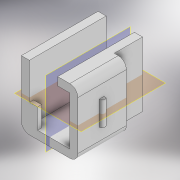
# Autodesk Inventor part: 부품1
Saved by Autodesk Inventor 2020 (Build 240168000, 168)
## iProperties
Created: 2022-04-05
Part Number: 부품1
Material: 일반
Document SubType Name: Modeling
Designer: Knowblesse
Density: 1 g/cm^3
Appearance: 기본값
Author: Knowblesse
## iProperties of the stored document _3D 인쇄.ipt
Created: 2022-04-05
Part Number: _3D 인쇄
Material: 일반
Document SubType Name: Modeling
Designer: Knowblesse
Density: 1 g/cm^3
Appearance: 기본값
Author: Knowblesse
Autodesk Inventor part; units mm, degrees
ref_plane "YZ Plane" through (0, 0, 0) normal (1, 0, 0) x (0, 1, 0)
ref_plane "XZ Plane" through (0, 0, 0) normal (0, 1, 0) x (-1, 0, 0)
ref_plane "XY Plane" through (0, 0, 0) normal (0, 0, 1) x (1, 0, 0)
sketch "스케치1" plane through (0, 0, 0) normal (0, 0, 1) x (1, 0, 0)
  line L0 (-3.5, -6) -> (3.5, -6)
  line L1 (3.5, -6) -> (3.5, 6)
  line L2 (3.5, 6) -> (-3.5, 6)
  line L3 (-3.5, 6) -> (-3.5, -6)
  line L4 (-3.5, -6) -> (3.5, 6) construction
  line L5 (3.5, -6) -> (-3.5, 6) construction
  line L6 (-5.5, 8) -> (-5.5, -8)
  line L7 (-5.5, -8) -> (5.5, -8)
  line L8 (5.5, -8) -> (5.5, 8)
  line L9 (5.5, 8) -> (3.5, 8)
  line L10 (3.5, 8) -> (3.5, 6)
  line L11 (-5.5, 8) -> (-3.5, 8)
  line L12 (-3.5, 8) -> (-3.5, 6)
  point P0 (0, 0)
  dimension "d0" = 7
  dimension "d1" = 12
  dimension "d2" = 2
  dimension "t" = 2
  dimension "d4" = 2
  dimension "d5" = 2
  constraints: 26 end point, 6 perpendicular, 2 midpoint, 2 parallel, 1 horizontal, 1 point on line, 1 vertical
  measures "d0" distance of L2.end L1.end
  measures "d1" distance of L1.end L0.end
  measures "d2" distance between parallel lines of L3 L6
  measures "t" distance between parallel lines of L8 L1
  measures "d4" distance between parallel lines of L0 L7
  measures "d5" distance between parallel lines of L11 L2
extrude "돌출1" add sketch "스케치1" along normal blind 7 contours L0 L1 L10 L9 L8 L7 L6 L11 L12 L3
sketch "스케치2" plane through (0, 0, 7) normal (0, 0, 1) x (1, 0, 0)
  line L0 (3.5, 8) -> (3.5, -6) projected
  line L1 (3.5, -6) -> (-3.5, -6) projected
  line L2 (-3.5, -6) -> (-3.5, 8) projected
  line L3 (-3.5, 8) -> (-5.5, 8) projected
  line L4 (-5.5, 8) -> (-5.5, -8) projected
  line L5 (-5.5, -8) -> (5.5, -8) projected
  line L6 (5.5, 8) -> (3.5, 8) projected
  line L7 (5.5, 8) -> (8.5, 8)
  line L8 (8.5, 8) -> (8.5, -8)
  line L9 (8.5, -8) -> (5.5, -8)
  point P0 (0, 0)
  dimension "d8" = 3
  constraints: 6 end point, 2 perpendicular, 1 horizontal
  measures "d8" distance of L8.end L5.end
extrude "돌출2" add sketch "스케치2" along normal blind 1
sketch "스케치3" plane through (0, 0, 8) normal (0, 0, 1) x (1, 0, 0)
  line L0 (-5.5, 8) -> (-5.5, -8) projected
  line L1 (-5.5, -8) -> (8.5, -8) projected
  line L2 (8.5, -8) -> (8.5, 8) projected
  line L3 (8.5, 8) -> (3.5, 8) projected
  line L4 (3.5, 8) -> (3.5, -6) projected
  line L5 (3.5, -6) -> (-3.5, -6) projected
  line L6 (-3.5, -6) -> (-3.5, 8) projected
  line L7 (-3.5, 8) -> (-5.5, 8) projected
  line L8 (3.5, -6) -> (-3.5, -6) projected
  line L9 (3.5, -6) -> (6.5, -6)
  line L10 (6.5, -6) -> (6.5, 6)
  line L11 (6.5, 6) -> (3.5, 6)
  line L12 (3.5, 8) -> (3.5, -6) projected
  point P0 (0, 0)
  dimension "d11" = 2
  dimension "d12" = 2
  constraints: 6 end point, 2 perpendicular, 1 horizontal, 1 point on line
  measures "d11" distance between parallel lines of L3 L11
  measures "d12" distance between parallel lines of L2 L10
extrude "돌출3" add sketch "스케치3" along normal blind 11 contours L7 L6 L5 L9 L10 L11 L4 L3 L2 L1 L0
sketch "스케치4" plane through (-3.5, -6, 0) normal (1, 0, 0) x (0, 0, -1)
  line L0 (-19, 0) -> (-19, 14) projected
  line L1 (0, 0) -> (-19, 0) projected
  line L2 (-19, 0) -> (-18, 0)
  line L3 (-18, 0) -> (-18, 5)
  line L4 (-18, 5) -> (-19, 5)
  line L5 (-19, 5) -> (-19, 0)
  point P0 (0, 6)
  dimension "d15" = 1
  dimension "d16" = 5
  constraints: 8 end point, 2 parallel, 1 horizontal, 1 perpendicular
  measures "d15" distance of L4.end L3.end
  measures "d16" distance of L3.end L2.end
extrude "돌출4" add sketch "스케치4" along normal blind 2
ref_plane "작업 평면1" through (-5.5, 0, 0) normal (0, 1, 0) x (1, 0, 0)
sketch "스케치5" plane through (-5.5, 0, 0) normal (0, 1, 0) x (1, 0, 0)
  line L0 (0, 0) -> (11, 0) projected
  line L1 (11, 0) -> (11, -7) projected
  line L2 (11, -7) -> (14, -7) projected
  line L3 (14, -7) -> (14, -19) projected
  line L4 (0, -19) -> (14, -19) projected
  line L5 (0, 0) -> (0, -19) projected
  line L6 (0, 0) -> (0, -19) projected
  circle A0 centre (0, -13) radius 0.7
  line L7 (-0.5217, -12.5333) -> (0, -12.5333)
  point P0 (5.5, 0)
  point P1 (0, -13.7)
  dimension "k" = 1.4
  dimension "d20" = 0.4667
  dimension "d21" = 6
  constraints: 2 end point, 2 point on line, 1 perpendicular, 3 other
  measures "d20" distance from line of point (0, -13) L7
  measures "d21" distance from line of L4 point (0, -13)
extrude "돌출5" add sketch "스케치5" along normal mid plane 6 contours L5 A0 L7 picked at (-0.0532, -13.305)
ref_plane "작업 평면2" through (1.5, -8, 0) normal (-1, 0, 0) x (0, 0, 1)
mirror "미러1" about plane through (1.5, -8, 0) normal (-1, 0, 0) of "돌출5"
fillet "모깎기1" radius 2 3 edges at (8.5, 8, 13) (-5.5, -8, 9.5) (8.5, -8, 13)
equation "\"d2\" = t"
equation "\"d4\" = t"
equation "\"d20\" = 0.333333 * k"
